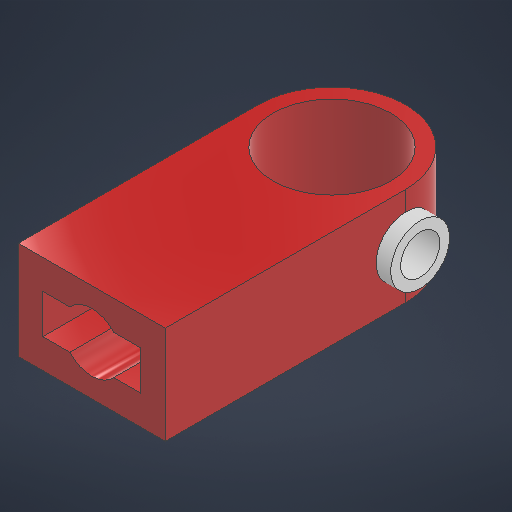
# Autodesk Inventor part: Link_OutsideV3
Saved by Autodesk Inventor 2025.1 (Build 291241000, 241)
## iProperties
Created: 2025-01-31
Part Number: Link_OutsideV3
Material: Generic
Document SubType Name: Modeling
Designer: m_kni
Density: 1 g/cm^3
Appearance: Default
Author: m_kni
Autodesk Inventor part; units mm, degrees
ref_plane "YZ Plane" through (0, 0, 0) normal (1, 0, 0) x (0, 1, 0)
ref_plane "XZ Plane" through (0, 0, 0) normal (0, 1, 0) x (-1, 0, 0)
ref_plane "XY Plane" through (0, 0, 0) normal (0, 0, 1) x (1, 0, 0)
sketch "Sketch1" plane through (0, 0, 0) normal (0, 1, 0) x (-1, 0, 0)
  line L0 (-0.0949, -0.0791) -> (-0.0949, -8.0791)
  circle A0 centre (-0.0949, -8.0791) radius 3
  line L1 (-0.0949, -0.0791) -> (-0.0949, 7.9209)
  circle A1 centre (-0.0949, 7.9209) radius 2.5
  circle A2 centre (-0.0949, 7.9209) radius 3.75
  circle A3 centre (-0.0949, -8.0791) radius 3.75
  line L2 (3.6551, 7.9209) -> (3.6551, -8.0791)
  line L3 (-3.8449, 7.9209) -> (-3.8449, -8.0791)
  line L4 (3.6551, 4.1709) -> (-3.8449, 4.1709)
  line L5 (3.6551, -4.3291) -> (-3.8449, -4.3291)
  point P0 (0, 0)
  dimension "d0" = 8
  dimension "d1" = 6
  dimension "d2" = 8
  dimension "d3" = 5
  dimension "d4" = 7.5
  dimension "d5" = 7.5
  constraints: 12 end point, 4 centre point, 4 coincident, 4 point on circle, 4 point on line, 4 vertical, 1 horizontal, 1 perpendicular, 1 tangent
  measures "d0" distance of L0.start L0.end
  measures "d1" diameter of A0
  measures "d2" distance of L0.start L1.end
  measures "d3" diameter of A1
  measures "d4" diameter of A2
  measures "d5" diameter of A3
extrude "Extrusion1" add sketch "Sketch1" along normal blind 5 contours L1 L4 L2 L5 L0 | L0 L5 L3 L4 L1 | L5 L2 A3 | A3 | A3 L3 L5
sketch "Sketch2" plane through (-3.6551, 0, 4.1709) normal (0, 0, 1) x (1, 0, 0)
  line L0 (0, 5) -> (7.5, 5) projected
  line L1 (0, 0) -> (7.5, 0)
  line L2 (7.5, 0) -> (7.5, 5)
  line L3 (7.5, 5) -> (0, 5)
  line L4 (0, 5) -> (0, 0)
  line L5 (7.5, 5) -> (0, 5)
  line L6 (0, 5) -> (0, 0)
  line L7 (0, 0) -> (7.5, 0)
  line L8 (7.5, 0) -> (7.5, 5)
  line L9 (7.5, 5) -> (0, 0) construction
  line L10 (0, 5) -> (7.5, 0) construction
  circle A0 centre (3.75, 2.5) radius 1.5
  line L11 (6.25, 3.5) -> (1.25, 3.5)
  line L12 (1.25, 3.5) -> (1.25, 1.5)
  line L13 (1.25, 1.5) -> (6.25, 1.5)
  line L14 (6.25, 1.5) -> (6.25, 3.5)
  line L15 (6.25, 3.5) -> (1.25, 1.5) construction
  line L16 (1.25, 3.5) -> (6.25, 1.5) construction
  point P0 (3.6551, 0)
  point P1 (4.868, 1.5)
  point P2 (4.868, 3.5)
  point P3 (2.632, 3.5)
  point P4 (2.632, 1.5)
  dimension "d8" = 3
  dimension "d9" = 5
  dimension "d10" = 2
  constraints: 32 end point, 6 parallel, 4 midpoint, 3 horizontal, 3 perpendicular, 1 centre point, 1 coincident
  measures "d8" diameter of A0
  measures "d9" distance of L13.end L12.end
  measures "d10" distance of L12.end L11.end
extrude "Extrusion2" cut sketch "Sketch2" against normal blind 8.5 contours A0 L13 L11 | A0 L11 L14 L13 | L11 A0 | A0 L13 | A0 L13 L12 L11
sketch "Sketch3" plane through (0, 5, 0) normal (0, 1, 0) x (1, 0, 0)
  line L0 (1.213, 4.3291) -> (2.5949, 4.3291) projected
  line L1 (-3.6551, -4.1709) -> (3.8449, -4.1709) projected
  point P0 (0, 0)
  dimension "d13" = 8.5
  measures "d13" distance between parallel lines of L0 L1
sketch "Sketch4" plane through (3.8449, 0, 4.1709) normal (1, 0, 0) x (0, 0, -1)
  line L0 (12.25, 0) -> (12.25, 5) projected
  circle A0 centre (12.25, 2.5) radius 1.5
  point P0 (4.1709, 0)
  dimension "d14" = 3
  constraints: 1 centre point, 1 coincident, 1 midpoint
  measures "d14" diameter of A0
extrude "Extrusion3" add sketch "Sketch4" along normal mid plane 1.5
sketch "Sketch5" plane through (4.5949, 2.5, -8.0791) normal (1, 0, 0) x (0, 0, -1)
  line L0 (0, -2.5) -> (0, 2.5) projected
  circle A0 centre (0, 0) radius 1
  point P0 (-8.0791, -2.5)
  dimension "d17" = 2
  constraints: 1 centre point, 1 midpoint
  measures "d17" diameter of A0
extrude "Extrusion4" cut sketch "Sketch5" against normal blind 3.0875
body "Solid1"
